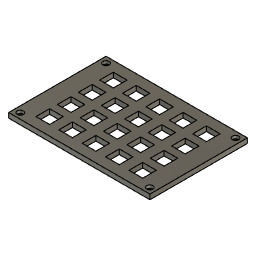
Front face v1 (Autodesk Fusion 360 design; units mm, degrees)
Autodesk Fusion 360 part; units mm, degrees
sketch "Esquisse1" plane through (0, 0, 0) normal (0, 0, 1) x (1, 0, 0)
  line L0 (0.1341, -76.3658) -> (64.4137, -0.1129)
  line L1 (64.4137, -0.1129) -> (129.0708, -76.1647)
  line L2 (129.0708, -76.1647) -> (129.0708, -86.1624)
  line L3 (0.1341, -76.133) -> (11.9451, -86.0425)
  line L4 (129.2084, -85.9931) -> (11.8004, -85.9931)
sketch "Esquisse2" plane through (-56.9768, 0, 48.0303) normal (-0.764582, 0, 0.644527) x (0, -1, 0)
  line L0 (-20.1587, 188.3406) -> (-20.1587, 88.7874)
  line L1 (-20.1587, 88.7874) -> (127.8413, 88.7874)
  line L2 (127.8413, 88.7874) -> (127.8413, 188.3406)
  line L3 (127.8413, 188.3406) -> (-20.1587, 188.3406)
  line L4 (-18.8236, 187.8236) -> (126.1751, 187.8236)
  line L5 (126.1751, 187.8236) -> (126.1751, 87.8252)
  line L6 (126.1751, 87.8252) -> (-18.8236, 87.8252)
  line L7 (-18.8236, 87.8252) -> (-18.8236, 187.8236)
  line L8 (-3.8235, 175.0777) -> (11.1766, 175.0777)
  line L9 (11.1766, 175.0777) -> (11.1766, 160.0776)
  line L10 (11.1766, 160.0776) -> (-3.8235, 160.0776)
  line L11 (-3.8235, 160.0776) -> (-3.8235, 175.0777)
  line L12 (21.1779, 175.0777) -> (36.178, 175.0777)
  line L13 (36.178, 175.0777) -> (36.178, 160.0776)
  line L14 (36.178, 160.0776) -> (21.1779, 160.0776)
  line L15 (21.1779, 160.0776) -> (21.1779, 175.0777)
  line L16 (46.1757, 175.0777) -> (61.1758, 175.0777)
  line L17 (61.1758, 175.0777) -> (61.1758, 160.0776)
  line L18 (61.1758, 160.0776) -> (46.1757, 160.0776)
  line L19 (46.1757, 160.0776) -> (46.1757, 175.0777)
  line L20 (71.1771, 175.0777) -> (86.1772, 175.0777)
  line L21 (86.1772, 175.0777) -> (86.1772, 160.0776)
  line L22 (86.1772, 160.0776) -> (71.1771, 160.0776)
  line L23 (71.1771, 160.0776) -> (71.1771, 175.0777)
  line L24 (96.1749, 175.0777) -> (111.175, 175.0777)
  line L25 (111.175, 175.0777) -> (111.175, 160.0776)
  line L26 (111.175, 160.0776) -> (96.1749, 160.0776)
  line L27 (96.1749, 160.0776) -> (96.1749, 175.0777)
  line L28 (-3.8235, 155.1387) -> (11.1766, 155.1387)
  line L29 (11.1766, 155.1387) -> (11.1766, 140.1386)
  line L30 (11.1766, 140.1386) -> (-3.8235, 140.1386)
  line L31 (-3.8235, 140.1386) -> (-3.8235, 155.1387)
  line L32 (21.1779, 155.1387) -> (36.178, 155.1387)
  line L33 (36.178, 155.1387) -> (36.178, 140.1386)
  line L34 (36.178, 140.1386) -> (21.1779, 140.1386)
  line L35 (21.1779, 140.1386) -> (21.1779, 155.1387)
  line L36 (46.1757, 155.1387) -> (61.1758, 155.1387)
  line L37 (61.1758, 155.1387) -> (61.1758, 140.1386)
  line L38 (61.1758, 140.1386) -> (46.1757, 140.1386)
  line L39 (46.1757, 140.1386) -> (46.1757, 155.1387)
  line L40 (71.1771, 155.1387) -> (86.1772, 155.1387)
  line L41 (86.1772, 155.1387) -> (86.1772, 140.1386)
  line L42 (86.1772, 140.1386) -> (71.1771, 140.1386)
  line L43 (71.1771, 140.1386) -> (71.1771, 155.1387)
  line L44 (96.1749, 155.1387) -> (111.175, 155.1387)
  line L45 (111.175, 155.1387) -> (111.175, 140.1386)
  line L46 (111.175, 140.1386) -> (96.1749, 140.1386)
  line L47 (96.1749, 140.1386) -> (96.1749, 155.1387)
  line L48 (-3.8235, 135.1997) -> (11.1766, 135.1997)
  line L49 (11.1766, 135.1997) -> (11.1766, 120.1996)
  line L50 (11.1766, 120.1996) -> (-3.8235, 120.1996)
  line L51 (-3.8235, 120.1996) -> (-3.8235, 135.1997)
  line L52 (21.1779, 135.1997) -> (36.178, 135.1997)
  line L53 (36.178, 135.1997) -> (36.178, 120.1996)
  line L54 (36.178, 120.1996) -> (21.1779, 120.1996)
  line L55 (21.1779, 120.1996) -> (21.1779, 135.1997)
  line L56 (46.1757, 135.1997) -> (61.1758, 135.1997)
  line L57 (61.1758, 135.1997) -> (61.1758, 120.1996)
  line L58 (61.1758, 120.1996) -> (46.1757, 120.1996)
  line L59 (46.1757, 120.1996) -> (46.1757, 135.1997)
  line L60 (71.1771, 135.1997) -> (86.1772, 135.1997)
  line L61 (86.1772, 135.1997) -> (86.1772, 120.1996)
  line L62 (86.1772, 120.1996) -> (71.1771, 120.1996)
  line L63 (71.1771, 120.1996) -> (71.1771, 135.1997)
  line L64 (96.1749, 135.1997) -> (111.175, 135.1997)
  line L65 (111.175, 135.1997) -> (111.175, 120.1996)
  line L66 (111.175, 120.1996) -> (96.1749, 120.1996)
  line L67 (96.1749, 120.1996) -> (96.1749, 135.1997)
  line L68 (-3.8235, 115.2643) -> (11.1766, 115.2643)
  line L69 (11.1766, 115.2643) -> (11.1766, 100.2642)
  line L70 (11.1766, 100.2642) -> (-3.8235, 100.2642)
  line L71 (-3.8235, 100.2642) -> (-3.8235, 115.2643)
  line L72 (21.1779, 115.2643) -> (36.178, 115.2643)
  line L73 (36.178, 115.2643) -> (36.178, 100.2642)
  line L74 (36.178, 100.2642) -> (21.1779, 100.2642)
  line L75 (21.1779, 100.2642) -> (21.1779, 115.2643)
  line L76 (46.1757, 115.2643) -> (61.1758, 115.2643)
  line L77 (61.1758, 115.2643) -> (61.1758, 100.2642)
  line L78 (61.1758, 100.2642) -> (46.1757, 100.2642)
  line L79 (46.1757, 100.2642) -> (46.1757, 115.2643)
  line L80 (71.1771, 115.2643) -> (86.1772, 115.2643)
  line L81 (86.1772, 115.2643) -> (86.1772, 100.2642)
  line L82 (86.1772, 100.2642) -> (71.1771, 100.2642)
  line L83 (71.1771, 100.2642) -> (71.1771, 115.2643)
  line L84 (96.1749, 115.2643) -> (111.175, 115.2643)
  line L85 (111.175, 115.2643) -> (111.175, 100.2642)
  line L86 (111.175, 100.2642) -> (96.1749, 100.2642)
  line L87 (96.1749, 100.2642) -> (96.1749, 115.2643)
sketch "Esquisse3" plane through (0, -127.8413, 0) normal (0, -1, 0) x (1, 0, 0)
  line L0 (3.7755, 116.2201) -> (64.4218, 188.1629)
  line L1 (64.4218, 188.1629) -> (126.5708, 115.0612)
  line L2 (126.5708, 115.0612) -> (126.5708, 108.6519)
  line L3 (126.5708, 108.6519) -> (12.796, 108.6519)
  line L4 (12.796, 108.6519) -> (3.7755, 116.2201)
  line L5 (0.249, 115.9156) -> (11.8862, 106.1519)
  line L6 (11.8862, 106.1519) -> (129.0708, 106.1519)
  line L7 (129.0708, 106.1519) -> (129.0708, 115.9803)
  line L8 (129.0708, 115.9803) -> (64.4137, 192.0321)
  line L9 (64.4137, 192.0321) -> (0.249, 115.9156)
  line L10 (64.4137, 192.0321) -> (0.249, 115.9156)
  line L11 (11.8862, 106.1519) -> (129.0708, 106.1519)
  line L12 (129.0708, 115.9803) -> (64.4137, 192.0321)
  constraint coincident L8.end L9.start
  constraint coincident L5.start L9.end
  constraint coincident L5.end L6.start
  constraint coincident L6.end L7.start
  constraint coincident L7.end L8.start
sketch "Esquisse4" plane through (0, 0, 0) normal (0, 0, 1) x (1, 0, 0)
  line L0 (155.2068, -87.1605) -> (155.2068, -101.1605)
  line L1 (165.2068, -65.4335) -> (179.2068, -65.4335)
  line L2 (141.2068, -65.4335) -> (155.2068, -65.4335)
  line L3 (165.2068, -79.4335) -> (165.2068, -65.4335)
  line L4 (107.7472, -87.1605) -> (107.7472, -101.1605)
  line L5 (203.2068, -101.1605) -> (189.2068, -101.1605)
  line L6 (93.7472, -101.1605) -> (93.7472, -87.1605)
  line L7 (93.7472, -79.4335) -> (93.7472, -65.4335)
  line L8 (117.2068, -87.1605) -> (131.2068, -87.1605)
  line L9 (189.2068, -79.4335) -> (189.2068, -65.4335)
  line L10 (179.2068, -79.4335) -> (165.2068, -79.4335)
  line L11 (165.2068, -87.1605) -> (179.2068, -87.1605)
  line L12 (155.2068, -101.1605) -> (141.2068, -101.1605)
  line L13 (93.7472, -87.1605) -> (107.7472, -87.1605)
  line L14 (93.7472, -65.4335) -> (107.7472, -65.4335)
  line L15 (141.2068, -79.4335) -> (141.2068, -65.4335)
  line L16 (155.2068, -79.4335) -> (141.2068, -79.4335)
  line L17 (131.2068, -101.1605) -> (117.2068, -101.1605)
  line L18 (117.2068, -101.1605) -> (117.2068, -87.1605)
  line L19 (131.2068, -65.4335) -> (131.2068, -79.4335)
  line L20 (165.2068, -101.1605) -> (165.2068, -87.1605)
  line L21 (189.2068, -65.4335) -> (203.2068, -65.4335)
  line L22 (141.2068, -101.1605) -> (141.2068, -87.1605)
  line L23 (107.7472, -101.1605) -> (93.7472, -101.1605)
  line L24 (131.2068, -79.4335) -> (117.2068, -79.4335)
  line L25 (141.2068, -87.1605) -> (155.2068, -87.1605)
  line L26 (131.2068, -87.1605) -> (131.2068, -101.1605)
  line L27 (155.2068, -65.4335) -> (155.2068, -79.4335)
  line L28 (107.7472, -65.4335) -> (107.7472, -79.4335)
  line L29 (203.2068, -79.4335) -> (189.2068, -79.4335)
  line L30 (179.2068, -101.1605) -> (165.2068, -101.1605)
  line L31 (179.2068, -87.1605) -> (179.2068, -101.1605)
  line L32 (203.2068, -65.4335) -> (203.2068, -79.4335)
  line L33 (179.2068, -65.4335) -> (179.2068, -79.4335)
  line L34 (117.2068, -79.4335) -> (117.2068, -65.4335)
  circle A0 centre (81.9919, -61.174) radius 1.8
  line L35 (164.9366, -144.6145) -> (164.9366, -130.6145)
  line L36 (107.7472, -79.4335) -> (93.7472, -79.4335)
  line L37 (117.2068, -65.4335) -> (131.2068, -65.4335)
  line L38 (155.2068, -122.8875) -> (141.2068, -122.8875)
  line L39 (178.9366, -130.6145) -> (178.9366, -144.6145)
  line L40 (140.9366, -130.6145) -> (154.9366, -130.6145)
  circle A1 centre (81.9919, -149.174) radius 1.8
  line L41 (220.8419, -155.024) -> (75.8419, -155.024)
  line L42 (188.9366, -144.6145) -> (188.9366, -130.6145)
  line L43 (189.2068, -108.8875) -> (203.2068, -108.8875)
  line L44 (179.2068, -122.8875) -> (165.2068, -122.8875)
  line L45 (130.9366, -144.6145) -> (116.9366, -144.6145)
  line L46 (107.477, -144.6145) -> (93.477, -144.6145)
  line L47 (165.2068, -108.8875) -> (179.2068, -108.8875)
  line L48 (140.9366, -144.6145) -> (140.9366, -130.6145)
  line L49 (189.2068, -87.1605) -> (203.2068, -87.1605)
  line L50 (93.477, -144.6145) -> (93.477, -130.6145)
  line L51 (130.9366, -130.6145) -> (130.9366, -144.6145)
  line L52 (116.9366, -130.6145) -> (130.9366, -130.6145)
  line L53 (75.8419, -55.024) -> (220.8419, -55.024)
  line L54 (141.2068, -108.8875) -> (155.2068, -108.8875)
  line L55 (179.2068, -108.8875) -> (179.2068, -122.8875)
  line L56 (107.7472, -122.8875) -> (93.7472, -122.8875)
  line L57 (75.8419, -155.024) -> (75.8419, -55.024)
  line L58 (93.7472, -122.8875) -> (93.7472, -108.8875)
  line L59 (107.477, -130.6145) -> (107.477, -144.6145)
  line L60 (220.8419, -55.024) -> (220.8419, -155.024)
  line L61 (202.9366, -144.6145) -> (188.9366, -144.6145)
  line L62 (117.2068, -122.8875) -> (117.2068, -108.8875)
  line L63 (117.2068, -108.8875) -> (131.2068, -108.8875)
  line L64 (164.9366, -130.6145) -> (178.9366, -130.6145)
  line L65 (141.2068, -122.8875) -> (141.2068, -108.8875)
  line L66 (154.9366, -130.6145) -> (154.9366, -144.6145)
  line L67 (202.9366, -130.6145) -> (202.9366, -144.6145)
  circle A2 centre (214.8129, -61.174) radius 1.8
  line L68 (203.2068, -108.8875) -> (203.2068, -122.8875)
  line L69 (203.2068, -122.8875) -> (189.2068, -122.8875)
  line L70 (93.7472, -108.8875) -> (107.7472, -108.8875)
  circle A3 centre (214.8129, -149.174) radius 1.8
  line L71 (203.2068, -87.1605) -> (203.2068, -101.1605)
  line L72 (189.2068, -101.1605) -> (189.2068, -87.1605)
  line L73 (189.2068, -122.8875) -> (189.2068, -108.8875)
  line L74 (155.2068, -108.8875) -> (155.2068, -122.8875)
  line L75 (116.9366, -144.6145) -> (116.9366, -130.6145)
  line L76 (188.9366, -130.6145) -> (202.9366, -130.6145)
  line L77 (165.2068, -122.8875) -> (165.2068, -108.8875)
  line L78 (131.2068, -108.8875) -> (131.2068, -122.8875)
  line L79 (154.9366, -144.6145) -> (140.9366, -144.6145)
  line L80 (93.477, -130.6145) -> (107.477, -130.6145)
  line L81 (107.7472, -108.8875) -> (107.7472, -122.8875)
  line L82 (131.2068, -122.8875) -> (117.2068, -122.8875)
  line L83 (178.9366, -144.6145) -> (164.9366, -144.6145)
extrude "Extrusion4" add sketch "Esquisse4" along normal blind 5
hole "Perçage2" at (81.9919, -61.174, 5) direction (0, 0, -1) diameter 3.6 depth 25 tip angle 180 counterbore diameter 6.4 counterbore depth 3
hole "Perçage3" at (81.9919, -149.174, 5) direction (0, 0, -1) diameter 3.6 depth 25 tip angle 180 counterbore diameter 6.4 counterbore depth 3
hole "Perçage4" at (214.8129, -149.174, 5) direction (0, 0, -1) diameter 3.6 depth 25 tip angle 180 counterbore diameter 6.4 counterbore depth 3
hole "Perçage5" at (214.8129, -61.174, 5) direction (0, 0, -1) diameter 3.6 depth 25 tip angle 180 counterbore diameter 6.4 counterbore depth 3
